Autodesk Fusion 360 part; units mm, degrees
(part 22 of 25)
sketch "Through Holes" plane through (0, 0, 0) normal (0, 0, 1) x (1, 0, 0)
  line L0 (72.5558, 49.13) -> (72.2242, 49.13)
  line L1 (72.2242, 49.13) -> (71.99, 49.3642)
  line L2 (72.7901, 49.6958) -> (72.7901, 49.3642)
  line L3 (72.2242, 49.9301) -> (72.5558, 49.9301)
  line L4 (74.53, 49.6958) -> (74.7642, 49.9301)
  line L5 (71.99, 49.3642) -> (71.99, 49.6958)
  arc A0 (68.1101, 6.35) -> (69.0499, 6.35) centre (68.58, 6.35) ccw
  line L6 (74.7642, 49.13) -> (74.53, 49.3642)
  line L7 (75.0958, 49.13) -> (74.7642, 49.13)
  line L8 (71.99, 49.6958) -> (72.2242, 49.9301)
  line L9 (74.7642, 49.9301) -> (75.0958, 49.9301)
  line L10 (72.2242, 49.9301) -> (72.5558, 49.9301)
  line L11 (74.53, 49.3642) -> (74.53, 49.6958)
  line L12 (75.0958, 49.13) -> (74.7642, 49.13)
  line L13 (75.3301, 49.3642) -> (75.0958, 49.13)
  line L14 (72.5558, 49.9301) -> (72.7901, 49.6958)
  arc A1 (66.5099, 6.35) -> (65.5701, 6.35) centre (66.04, 6.35) ccw
  line L15 (72.7901, 49.3642) -> (72.5558, 49.13)
  line L16 (74.7642, 49.9301) -> (75.0958, 49.9301)
  line L17 (74.7642, 49.13) -> (74.53, 49.3642)
  line L18 (72.7901, 49.3642) -> (72.5558, 49.13)
  line L19 (72.2242, 49.13) -> (71.99, 49.3642)
  line L20 (71.99, 49.3642) -> (71.99, 49.6958)
  line L21 (74.53, 49.6958) -> (74.7642, 49.9301)
  line L22 (71.99, 49.3642) -> (71.99, 49.6958)
  line L23 (75.3301, 49.3642) -> (75.0958, 49.13)
  line L24 (53.1558, 17.3355) -> (52.8955, 17.5958)
  line L25 (53.7845, 17.5958) -> (53.5242, 17.3355)
  arc A2 (50.8, 18.2245) -> (50.8, 17.3355) centre (50.8, 17.78) ccw
  line L26 (53.5242, 17.3355) -> (53.1558, 17.3355)
  line L27 (74.53, 49.3642) -> (74.53, 49.6958)
  arc A3 (50.8, 17.3355) -> (50.8, 18.2245) centre (50.8, 17.78) ccw
  line L28 (53.1558, 18.2245) -> (53.5242, 18.2245)
  arc A4 (50.8, 18.2245) -> (50.8, 17.3355) centre (50.8, 17.78) ccw
  line L29 (72.7901, 49.6958) -> (72.7901, 49.3642)
  line L30 (75.3301, 49.6958) -> (75.3301, 49.3642)
  line L31 (53.5242, 18.2245) -> (53.7845, 17.9642)
  line L32 (52.8955, 17.5958) -> (52.8955, 17.9642)
  line L33 (52.8955, 17.9642) -> (53.1558, 18.2245)
  arc A5 (65.5701, 6.35) -> (66.5099, 6.35) centre (66.04, 6.35) ccw
  line L34 (74.53, 49.3642) -> (74.53, 49.6958)
  arc A6 (69.0499, 6.35) -> (68.1101, 6.35) centre (68.58, 6.35) ccw
  line L35 (74.53, 49.3642) -> (74.53, 49.6958)
  line L36 (72.5558, 49.13) -> (72.2242, 49.13)
  line L37 (75.3301, 49.6958) -> (75.3301, 49.3642)
  line L38 (71.99, 49.6958) -> (72.2242, 49.9301)
  line L39 (72.5558, 49.9301) -> (72.7901, 49.6958)
  line L40 (52.8955, 17.5958) -> (52.8955, 17.9642)
  line L41 (75.0958, 49.9301) -> (75.3301, 49.6958)
  line L42 (75.0958, 49.9301) -> (75.3301, 49.6958)
  line L43 (71.99, 49.3642) -> (71.99, 49.6958)
  arc A7 (61.4299, 6.35) -> (60.4901, 6.35) centre (60.96, 6.35) ccw
  arc A8 (40.1701, 6.35) -> (41.1099, 6.35) centre (40.64, 6.35) ccw
  arc A9 (57.9501, 6.35) -> (58.8899, 6.35) centre (58.42, 6.35) ccw
  arc A10 (14.3891, 33.909) -> (13.5509, 33.909) centre (13.97, 33.909) ccw
  arc A11 (4.318, 50.3555) -> (4.318, 53.5305) centre (4.318, 51.943) ccw
  arc A12 (14.3891, 44.069) -> (13.5509, 44.069) centre (13.97, 44.069) ccw
  arc A13 (50.8, 17.3355) -> (50.8, 18.2245) centre (50.8, 17.78) ccw
  arc A14 (33.4899, 6.35) -> (32.5501, 6.35) centre (33.02, 6.35) ccw
  arc A15 (50.3301, 6.35) -> (51.2699, 6.35) centre (50.8, 6.35) ccw
  arc A16 (41.1099, 6.35) -> (40.1701, 6.35) centre (40.64, 6.35) ccw
  arc A17 (45.2501, 6.35) -> (46.1899, 6.35) centre (45.72, 6.35) ccw
  arc A18 (61.4299, 6.35) -> (60.4901, 6.35) centre (60.96, 6.35) ccw
  arc A19 (4.318, 50.3555) -> (4.318, 53.5305) centre (4.318, 51.943) ccw
  arc A20 (45.2501, 6.35) -> (46.1899, 6.35) centre (45.72, 6.35) ccw
  arc A21 (40.1701, 6.35) -> (41.1099, 6.35) centre (40.64, 6.35) ccw
  arc A22 (63.9699, 6.35) -> (63.0301, 6.35) centre (63.5, 6.35) ccw
  arc A23 (66.5099, 6.35) -> (65.5701, 6.35) centre (66.04, 6.35) ccw
  arc A24 (13.5509, 33.909) -> (14.3891, 33.909) centre (13.97, 33.909) ccw
  arc A25 (14.3891, 44.069) -> (13.5509, 44.069) centre (13.97, 44.069) ccw
  arc A26 (80.645, 50.3555) -> (80.645, 53.5305) centre (80.645, 51.943) ccw
  arc A27 (58.8899, 6.35) -> (57.9501, 6.35) centre (58.42, 6.35) ccw
  arc A28 (68.1101, 6.35) -> (69.0499, 6.35) centre (68.58, 6.35) ccw
  arc A29 (37.6301, 6.35) -> (38.5699, 6.35) centre (38.1, 6.35) ccw
  arc A30 (35.0901, 6.35) -> (36.0299, 6.35) centre (35.56, 6.35) ccw
  line L44 (53.1558, 18.2245) -> (53.5242, 18.2245)
  arc A31 (14.3891, 33.909) -> (13.5509, 33.909) centre (13.97, 33.909) ccw
  arc A32 (13.5509, 44.069) -> (14.3891, 44.069) centre (13.97, 44.069) ccw
  arc A33 (32.5501, 6.35) -> (33.4899, 6.35) centre (33.02, 6.35) ccw
  arc A34 (50.3301, 6.35) -> (51.2699, 6.35) centre (50.8, 6.35) ccw
  line L45 (53.7845, 17.5958) -> (53.5242, 17.3355)
  arc A35 (38.5699, 6.35) -> (37.6301, 6.35) centre (38.1, 6.35) ccw
  arc A36 (4.318, 53.5305) -> (4.318, 50.3555) centre (4.318, 51.943) ccw
  arc A37 (43.6499, 6.35) -> (42.7101, 6.35) centre (43.18, 6.35) ccw
  arc A38 (60.4901, 6.35) -> (61.4299, 6.35) centre (60.96, 6.35) ccw
  arc A39 (56.3499, 6.35) -> (55.4101, 6.35) centre (55.88, 6.35) ccw
  arc A40 (69.0499, 6.35) -> (68.1101, 6.35) centre (68.58, 6.35) ccw
  line L46 (52.8955, 17.5958) -> (52.8955, 17.9642)
  arc A41 (13.5509, 33.909) -> (14.3891, 33.909) centre (13.97, 33.909) ccw
  arc A42 (47.7901, 6.35) -> (48.7299, 6.35) centre (48.26, 6.35) ccw
  line L47 (53.5242, 17.3355) -> (53.1558, 17.3355)
  arc A43 (65.5701, 6.35) -> (66.5099, 6.35) centre (66.04, 6.35) ccw
  arc A44 (42.7101, 6.35) -> (43.6499, 6.35) centre (43.18, 6.35) ccw
  arc A45 (63.0301, 6.35) -> (63.9699, 6.35) centre (63.5, 6.35) ccw
  arc A46 (80.645, 53.5305) -> (80.645, 50.3555) centre (80.645, 51.943) ccw
  line L48 (53.7845, 17.9642) -> (53.7845, 17.5958)
  arc A47 (42.7101, 6.35) -> (43.6499, 6.35) centre (43.18, 6.35) ccw
  arc A48 (38.5699, 6.35) -> (37.6301, 6.35) centre (38.1, 6.35) ccw
  arc A49 (56.3499, 6.35) -> (55.4101, 6.35) centre (55.88, 6.35) ccw
  line L49 (52.8955, 17.5958) -> (52.8955, 17.9642)
  arc A50 (4.318, 53.5305) -> (4.318, 50.3555) centre (4.318, 51.943) ccw
  arc A51 (80.645, 50.3555) -> (80.645, 53.5305) centre (80.645, 51.943) ccw
  arc A52 (48.7299, 6.35) -> (47.7901, 6.35) centre (48.26, 6.35) ccw
  arc A53 (33.4899, 6.35) -> (32.5501, 6.35) centre (33.02, 6.35) ccw
  line L50 (52.8955, 17.9642) -> (53.1558, 18.2245)
  arc A54 (36.0299, 6.35) -> (35.0901, 6.35) centre (35.56, 6.35) ccw
  line L51 (53.1558, 17.3355) -> (52.8955, 17.5958)
  arc A55 (32.5501, 6.35) -> (33.4899, 6.35) centre (33.02, 6.35) ccw
  arc A56 (13.5509, 44.069) -> (14.3891, 44.069) centre (13.97, 44.069) ccw
  arc A57 (51.2699, 6.35) -> (50.3301, 6.35) centre (50.8, 6.35) ccw
  arc A58 (43.6499, 6.35) -> (42.7101, 6.35) centre (43.18, 6.35) ccw
  arc A59 (37.6301, 6.35) -> (38.5699, 6.35) centre (38.1, 6.35) ccw
  line L52 (53.5242, 18.2245) -> (53.7845, 17.9642)
  line L53 (53.7845, 17.9642) -> (53.7845, 17.5958)
  arc A60 (80.645, 53.5305) -> (80.645, 50.3555) centre (80.645, 51.943) ccw
  line L54 (40.7768, 32.6898) -> (40.5032, 32.6898)
  line L55 (50.4698, 32.8832) -> (50.4698, 33.1568)
  line L56 (40.3098, 32.8832) -> (40.3098, 33.1568)
  line L57 (40.9702, 32.8832) -> (40.7768, 32.6898)
  line L58 (51.1302, 33.1568) -> (51.1302, 32.8832)
  line L59 (40.9702, 32.8832) -> (40.7768, 32.6898)
  arc A61 (57.9501, 6.35) -> (58.8899, 6.35) centre (58.42, 6.35) ccw
  arc A62 (60.4901, 6.35) -> (61.4299, 6.35) centre (60.96, 6.35) ccw
  line L60 (51.1302, 32.8832) -> (50.9368, 32.6898)
  line L61 (50.6632, 32.6898) -> (50.4698, 32.8832)
  line L62 (40.5032, 32.6898) -> (40.3098, 32.8832)
  line L63 (50.4698, 33.1568) -> (50.6632, 33.3502)
  line L64 (50.6632, 33.3502) -> (50.9368, 33.3502)
  line L65 (50.9368, 33.3502) -> (51.1302, 33.1568)
  line L66 (51.1302, 33.1568) -> (51.1302, 32.8832)
  line L67 (40.3098, 33.1568) -> (40.5032, 33.3502)
  arc A63 (56.3499, 49.53) -> (55.4101, 49.53) centre (55.88, 49.53) ccw
  arc A64 (47.7901, 6.35) -> (48.7299, 6.35) centre (48.26, 6.35) ccw
  arc A65 (63.9699, 6.35) -> (63.0301, 6.35) centre (63.5, 6.35) ccw
  arc A66 (61.4299, 49.53) -> (60.4901, 49.53) centre (60.96, 49.53) ccw
  arc A67 (57.9501, 49.53) -> (58.8899, 49.53) centre (58.42, 49.53) ccw
  arc A68 (55.4101, 49.53) -> (56.3499, 49.53) centre (55.88, 49.53) ccw
  line L68 (40.9702, 33.1568) -> (40.9702, 32.8832)
  arc A69 (53.8099, 6.35) -> (52.8701, 6.35) centre (53.34, 6.35) ccw
  line L69 (40.5032, 32.6898) -> (40.3098, 32.8832)
  arc A70 (55.4101, 6.35) -> (56.3499, 6.35) centre (55.88, 6.35) ccw
  arc A71 (60.4901, 49.53) -> (61.4299, 49.53) centre (60.96, 49.53) ccw
  arc A72 (46.1899, 6.35) -> (45.2501, 6.35) centre (45.72, 6.35) ccw
  arc A73 (58.8899, 49.53) -> (57.9501, 49.53) centre (58.42, 49.53) ccw
  line L70 (50.9368, 32.6898) -> (50.6632, 32.6898)
  line L71 (40.9702, 33.1568) -> (40.9702, 32.8832)
  arc A74 (36.0299, 6.35) -> (35.0901, 6.35) centre (35.56, 6.35) ccw
  arc A75 (55.4101, 49.53) -> (56.3499, 49.53) centre (55.88, 49.53) ccw
  arc A76 (53.8099, 49.53) -> (52.8701, 49.53) centre (53.34, 49.53) ccw
  arc A77 (35.0901, 6.35) -> (36.0299, 6.35) centre (35.56, 6.35) ccw
  line L72 (40.5032, 33.3502) -> (40.7768, 33.3502)
  arc A78 (48.7299, 6.35) -> (47.7901, 6.35) centre (48.26, 6.35) ccw
  line L73 (50.6632, 32.6898) -> (50.4698, 32.8832)
  line L74 (40.3098, 32.8832) -> (40.3098, 33.1568)
  arc A79 (52.8701, 6.35) -> (53.8099, 6.35) centre (53.34, 6.35) ccw
  line L75 (50.4698, 33.1568) -> (50.6632, 33.3502)
  arc A80 (58.8899, 6.35) -> (57.9501, 6.35) centre (58.42, 6.35) ccw
  line L76 (40.5032, 33.3502) -> (40.7768, 33.3502)
  line L77 (40.3098, 33.1568) -> (40.5032, 33.3502)
  line L78 (40.9702, 33.1568) -> (40.9702, 32.8832)
  line L79 (40.7768, 33.3502) -> (40.9702, 33.1568)
  line L80 (40.7768, 33.3502) -> (40.9702, 33.1568)
  line L81 (40.7768, 32.6898) -> (40.5032, 32.6898)
  arc A81 (46.1899, 6.35) -> (45.2501, 6.35) centre (45.72, 6.35) ccw
  line L82 (50.6632, 33.3502) -> (50.9368, 33.3502)
  arc A82 (55.4101, 6.35) -> (56.3499, 6.35) centre (55.88, 6.35) ccw
  arc A83 (41.1099, 6.35) -> (40.1701, 6.35) centre (40.64, 6.35) ccw
  arc A84 (52.8701, 6.35) -> (53.8099, 6.35) centre (53.34, 6.35) ccw
  line L83 (50.9368, 33.3502) -> (51.1302, 33.1568)
  line L84 (51.1302, 32.8832) -> (50.9368, 32.6898)
  arc A85 (53.8099, 6.35) -> (52.8701, 6.35) centre (53.34, 6.35) ccw
  line L85 (51.1302, 33.1568) -> (51.1302, 32.8832)
  line L86 (51.1302, 33.1568) -> (51.1302, 32.8832)
  line L87 (40.9702, 33.1568) -> (40.9702, 32.8832)
  arc A86 (51.2699, 6.35) -> (50.3301, 6.35) centre (50.8, 6.35) ccw
  arc A87 (63.0301, 6.35) -> (63.9699, 6.35) centre (63.5, 6.35) ccw
  line L88 (50.9368, 32.6898) -> (50.6632, 32.6898)
  line L89 (50.4698, 32.8832) -> (50.4698, 33.1568)
  arc A88 (42.7101, 49.53) -> (43.6499, 49.53) centre (43.18, 49.53) ccw
  arc A89 (24.9301, 49.53) -> (25.8699, 49.53) centre (25.4, 49.53) ccw
  arc A90 (28.7401, 24.4602) -> (29.6799, 24.4602) centre (29.21, 24.4602) ccw
  arc A91 (51.2699, 49.53) -> (50.3301, 49.53) centre (50.8, 49.53) ccw
  arc A92 (33.8201, 24.4602) -> (34.7599, 24.4602) centre (34.29, 24.4602) ccw
  line L90 (29.21, 24.4602) -> (29.21, 26.3398)
  line L91 (36.83, 24.4602) -> (36.83, 26.3398)
  arc A93 (28.4099, 49.53) -> (27.4701, 49.53) centre (27.94, 49.53) ccw
  arc A94 (46.1899, 49.53) -> (45.2501, 49.53) centre (45.72, 49.53) ccw
  arc A95 (52.8701, 49.53) -> (53.8099, 49.53) centre (53.34, 49.53) ccw
  line L92 (34.29, 24.4602) -> (34.29, 26.3398)
  line L93 (31.75, 24.4602) -> (31.75, 26.3398)
  arc A96 (60.4901, 49.53) -> (61.4299, 49.53) centre (60.96, 49.53) ccw
  arc A97 (51.2699, 49.53) -> (50.3301, 49.53) centre (50.8, 49.53) ccw
  arc A98 (37.6301, 49.53) -> (38.5699, 49.53) centre (38.1, 49.53) ccw
  arc A99 (38.5699, 49.53) -> (37.6301, 49.53) centre (38.1, 49.53) ccw
  arc A100 (26.2001, 24.4602) -> (27.1399, 24.4602) centre (26.67, 24.4602) ccw
  arc A101 (30.9499, 49.53) -> (30.0101, 49.53) centre (30.48, 49.53) ccw
  arc A102 (24.9301, 49.53) -> (25.8699, 49.53) centre (25.4, 49.53) ccw
  arc A103 (48.7299, 49.53) -> (47.7901, 49.53) centre (48.26, 49.53) ccw
  arc A104 (32.5501, 49.53) -> (33.4899, 49.53) centre (33.02, 49.53) ccw
  arc A105 (25.8699, 49.53) -> (24.9301, 49.53) centre (25.4, 49.53) ccw
  arc A106 (37.6301, 49.53) -> (38.5699, 49.53) centre (38.1, 49.53) ccw
  arc A107 (30.0101, 49.53) -> (30.9499, 49.53) centre (30.48, 49.53) ccw
  arc A108 (45.2501, 49.53) -> (46.1899, 49.53) centre (45.72, 49.53) ccw
  arc A109 (43.6499, 49.53) -> (42.7101, 49.53) centre (43.18, 49.53) ccw
  arc A110 (41.1099, 49.53) -> (40.1701, 49.53) centre (40.64, 49.53) ccw
  arc A111 (50.3301, 49.53) -> (51.2699, 49.53) centre (50.8, 49.53) ccw
  arc A112 (48.7299, 49.53) -> (47.7901, 49.53) centre (48.26, 49.53) ccw
  arc A113 (57.9501, 49.53) -> (58.8899, 49.53) centre (58.42, 49.53) ccw
  arc A114 (25.8699, 49.53) -> (24.9301, 49.53) centre (25.4, 49.53) ccw
  arc A115 (43.6499, 49.53) -> (42.7101, 49.53) centre (43.18, 49.53) ccw
  arc A116 (47.7901, 49.53) -> (48.7299, 49.53) centre (48.26, 49.53) ccw
  arc A117 (56.3499, 49.53) -> (55.4101, 49.53) centre (55.88, 49.53) ccw
  arc A118 (28.4099, 49.53) -> (27.4701, 49.53) centre (27.94, 49.53) ccw
  arc A119 (27.4701, 49.53) -> (28.4099, 49.53) centre (27.94, 49.53) ccw
  arc A120 (46.1899, 49.53) -> (45.2501, 49.53) centre (45.72, 49.53) ccw
  arc A121 (32.5501, 49.53) -> (33.4899, 49.53) centre (33.02, 49.53) ccw
  arc A122 (45.2501, 49.53) -> (46.1899, 49.53) centre (45.72, 49.53) ccw
  arc A123 (33.4899, 49.53) -> (32.5501, 49.53) centre (33.02, 49.53) ccw
  arc A124 (61.4299, 49.53) -> (60.4901, 49.53) centre (60.96, 49.53) ccw
  arc A125 (30.9499, 49.53) -> (30.0101, 49.53) centre (30.48, 49.53) ccw
  arc A126 (42.7101, 49.53) -> (43.6499, 49.53) centre (43.18, 49.53) ccw
  arc A127 (40.1701, 49.53) -> (41.1099, 49.53) centre (40.64, 49.53) ccw
  arc A128 (30.0101, 49.53) -> (30.9499, 49.53) centre (30.48, 49.53) ccw
  arc A129 (38.5699, 49.53) -> (37.6301, 49.53) centre (38.1, 49.53) ccw
  arc A130 (35.0901, 49.53) -> (36.0299, 49.53) centre (35.56, 49.53) ccw
  arc A131 (41.1099, 49.53) -> (40.1701, 49.53) centre (40.64, 49.53) ccw
  line L94 (26.67, 24.4602) -> (26.67, 26.3398)
  arc A132 (58.8899, 49.53) -> (57.9501, 49.53) centre (58.42, 49.53) ccw
  arc A133 (33.4899, 49.53) -> (32.5501, 49.53) centre (33.02, 49.53) ccw
  arc A134 (53.8099, 49.53) -> (52.8701, 49.53) centre (53.34, 49.53) ccw
  arc A135 (36.0299, 49.53) -> (35.0901, 49.53) centre (35.56, 49.53) ccw
  arc A136 (28.7401, 24.4602) -> (29.6799, 24.4602) centre (29.21, 24.4602) ccw
  line L95 (29.21, 24.4602) -> (29.21, 26.3398)
  arc A137 (47.7901, 49.53) -> (48.7299, 49.53) centre (48.26, 49.53) ccw
  arc A138 (27.4701, 49.53) -> (28.4099, 49.53) centre (27.94, 49.53) ccw
  arc A139 (35.0901, 49.53) -> (36.0299, 49.53) centre (35.56, 49.53) ccw
  arc A140 (36.0299, 49.53) -> (35.0901, 49.53) centre (35.56, 49.53) ccw
  arc A141 (50.3301, 49.53) -> (51.2699, 49.53) centre (50.8, 49.53) ccw
  arc A142 (40.1701, 49.53) -> (41.1099, 49.53) centre (40.64, 49.53) ccw
  arc A143 (34.7599, 26.3398) -> (33.8201, 26.3398) centre (34.29, 26.3398) ccw
  arc A144 (52.8701, 49.53) -> (53.8099, 49.53) centre (53.34, 49.53) ccw
  arc A145 (27.1399, 26.3398) -> (26.2001, 26.3398) centre (26.67, 26.3398) ccw
  arc A146 (27.1399, 26.3398) -> (26.2001, 26.3398) centre (26.67, 26.3398) ccw
  arc A147 (36.3601, 24.4602) -> (37.2999, 24.4602) centre (36.83, 24.4602) ccw
  arc A148 (29.6799, 26.3398) -> (28.7401, 26.3398) centre (29.21, 26.3398) ccw
  line L96 (31.75, 24.4602) -> (31.75, 26.3398)
  arc A149 (37.2999, 26.3398) -> (36.3601, 26.3398) centre (36.83, 26.3398) ccw
  arc A150 (29.6799, 26.3398) -> (28.7401, 26.3398) centre (29.21, 26.3398) ccw
  arc A151 (31.2801, 24.4602) -> (32.2199, 24.4602) centre (31.75, 24.4602) ccw
  line L97 (34.29, 24.4602) -> (34.29, 26.3398)
  arc A152 (34.7599, 26.3398) -> (33.8201, 26.3398) centre (34.29, 26.3398) ccw
  arc A153 (26.2001, 24.4602) -> (27.1399, 24.4602) centre (26.67, 24.4602) ccw
  arc A154 (31.2801, 24.4602) -> (32.2199, 24.4602) centre (31.75, 24.4602) ccw
  line L98 (26.67, 24.4602) -> (26.67, 26.3398)
  arc A155 (32.2199, 26.3398) -> (31.2801, 26.3398) centre (31.75, 26.3398) ccw
  arc A156 (37.2999, 26.3398) -> (36.3601, 26.3398) centre (36.83, 26.3398) ccw
  arc A157 (74.1299, 32.6898) -> (73.1901, 32.6898) centre (73.66, 32.6898) ccw
  line L99 (78.74, 43.5102) -> (78.74, 45.3898)
  line L100 (76.2, 30.8102) -> (76.2, 32.6898)
  arc A158 (81.7499, 45.3898) -> (80.8101, 45.3898) centre (81.28, 45.3898) ccw
  arc A159 (79.2099, 45.3898) -> (78.2701, 45.3898) centre (78.74, 45.3898) ccw
  arc A160 (73.1901, 43.5102) -> (74.1299, 43.5102) centre (73.66, 43.5102) ccw
  line L101 (73.66, 43.5102) -> (73.66, 45.3898)
  line L102 (36.83, 24.4602) -> (36.83, 26.3398)
  line L103 (76.2, 43.5102) -> (76.2, 45.3898)
  arc A161 (81.7499, 45.3898) -> (80.8101, 45.3898) centre (81.28, 45.3898) ccw
  line L104 (78.74, 30.8102) -> (78.74, 32.6898)
  arc A162 (80.8101, 43.5102) -> (81.7499, 43.5102) centre (81.28, 43.5102) ccw
  arc A163 (73.1901, 30.8102) -> (74.1299, 30.8102) centre (73.66, 30.8102) ccw
  arc A164 (33.8201, 24.4602) -> (34.7599, 24.4602) centre (34.29, 24.4602) ccw
  arc A165 (79.2099, 45.3898) -> (78.2701, 45.3898) centre (78.74, 45.3898) ccw
  arc A166 (76.6699, 45.3898) -> (75.7301, 45.3898) centre (76.2, 45.3898) ccw
  arc A167 (76.6699, 45.3898) -> (75.7301, 45.3898) centre (76.2, 45.3898) ccw
  line L105 (73.66, 30.8102) -> (73.66, 32.6898)
  arc A168 (75.7301, 30.8102) -> (76.6699, 30.8102) centre (76.2, 30.8102) ccw
  line L106 (81.28, 43.5102) -> (81.28, 45.3898)
  line L107 (73.66, 30.8102) -> (73.66, 32.6898)
  arc A169 (74.1299, 45.3898) -> (73.1901, 45.3898) centre (73.66, 45.3898) ccw
  line L108 (73.66, 43.5102) -> (73.66, 45.3898)
  arc A170 (76.6699, 32.6898) -> (75.7301, 32.6898) centre (76.2, 32.6898) ccw
  arc A171 (75.7301, 30.8102) -> (76.6699, 30.8102) centre (76.2, 30.8102) ccw
  arc A172 (73.1901, 30.8102) -> (74.1299, 30.8102) centre (73.66, 30.8102) ccw
  arc A173 (78.2701, 43.5102) -> (79.2099, 43.5102) centre (78.74, 43.5102) ccw
  arc A174 (76.6699, 32.6898) -> (75.7301, 32.6898) centre (76.2, 32.6898) ccw
  arc A175 (74.1299, 45.3898) -> (73.1901, 45.3898) centre (73.66, 45.3898) ccw
  arc A176 (75.7301, 43.5102) -> (76.6699, 43.5102) centre (76.2, 43.5102) ccw
  arc A177 (75.7301, 43.5102) -> (76.6699, 43.5102) centre (76.2, 43.5102) ccw
  line L109 (76.2, 30.8102) -> (76.2, 32.6898)
  arc A178 (80.8101, 43.5102) -> (81.7499, 43.5102) centre (81.28, 43.5102) ccw
  arc A179 (36.3601, 24.4602) -> (37.2999, 24.4602) centre (36.83, 24.4602) ccw
  line L110 (81.28, 43.5102) -> (81.28, 45.3898)
  arc A180 (74.1299, 32.6898) -> (73.1901, 32.6898) centre (73.66, 32.6898) ccw
  arc A181 (78.2701, 43.5102) -> (79.2099, 43.5102) centre (78.74, 43.5102) ccw
  arc A182 (73.1901, 43.5102) -> (74.1299, 43.5102) centre (73.66, 43.5102) ccw
  arc A183 (32.2199, 26.3398) -> (31.2801, 26.3398) centre (31.75, 26.3398) ccw
  line L111 (78.74, 43.5102) -> (78.74, 45.3898)
  line L112 (76.2, 43.5102) -> (76.2, 45.3898)
  line L113 (63.5, 42.2402) -> (63.5, 44.1198)
  arc A184 (58.8899, 44.1198) -> (57.9501, 44.1198) centre (58.42, 44.1198) ccw
  line L114 (27.0701, 37.9342) -> (26.8358, 37.7)
  arc A185 (65.5701, 42.2402) -> (66.5099, 42.2402) centre (66.04, 42.2402) ccw
  line L115 (34.4558, 37.7) -> (34.1242, 37.7)
  line L116 (26.5042, 37.7) -> (26.27, 37.9342)
  arc A186 (81.7499, 32.6898) -> (80.8101, 32.6898) centre (81.28, 32.6898) ccw
  line L117 (66.04, 42.2402) -> (66.04, 44.1198)
  line L118 (63.5, 42.2402) -> (63.5, 44.1198)
  arc A187 (60.4901, 42.2402) -> (61.4299, 42.2402) centre (60.96, 42.2402) ccw
  arc A188 (66.5099, 44.1198) -> (65.5701, 44.1198) centre (66.04, 44.1198) ccw
  line L119 (33.89, 37.9342) -> (33.89, 38.2658)
  line L120 (34.1242, 37.7) -> (33.89, 37.9342)
  line L121 (34.69, 38.2658) -> (34.69, 37.9342)
  line L122 (34.69, 37.9342) -> (34.4558, 37.7)
  line L123 (34.4558, 37.7) -> (34.1242, 37.7)
  line L124 (34.69, 38.2658) -> (34.69, 37.9342)
  line L125 (34.1242, 38.5001) -> (34.4558, 38.5001)
  arc A189 (63.9699, 44.1198) -> (63.0301, 44.1198) centre (63.5, 44.1198) ccw
  line L126 (81.28, 30.8102) -> (81.28, 32.6898)
  arc A190 (80.8101, 30.8102) -> (81.7499, 30.8102) centre (81.28, 30.8102) ccw
  arc A191 (65.5701, 42.2402) -> (66.5099, 42.2402) centre (66.04, 42.2402) ccw
  arc A192 (65.5701, 30.8102) -> (66.5099, 30.8102) centre (66.04, 30.8102) ccw
  arc A193 (61.4299, 32.6898) -> (60.4901, 32.6898) centre (60.96, 32.6898) ccw
  line L127 (66.04, 42.2402) -> (66.04, 44.1198)
  arc A194 (63.9699, 44.1198) -> (63.0301, 44.1198) centre (63.5, 44.1198) ccw
  arc A195 (63.0301, 42.2402) -> (63.9699, 42.2402) centre (63.5, 42.2402) ccw
  arc A196 (79.2099, 32.6898) -> (78.2701, 32.6898) centre (78.74, 32.6898) ccw
  line L128 (26.8358, 37.7) -> (26.5042, 37.7)
  arc A197 (81.7499, 32.6898) -> (80.8101, 32.6898) centre (81.28, 32.6898) ccw
  arc A198 (63.0301, 30.8102) -> (63.9699, 30.8102) centre (63.5, 30.8102) ccw
  line L129 (34.69, 38.2658) -> (34.69, 37.9342)
  line L130 (34.4558, 38.5001) -> (34.69, 38.2658)
  arc A199 (60.4901, 42.2402) -> (61.4299, 42.2402) centre (60.96, 42.2402) ccw
  arc A200 (63.0301, 30.8102) -> (63.9699, 30.8102) centre (63.5, 30.8102) ccw
  arc A201 (61.4299, 44.1198) -> (60.4901, 44.1198) centre (60.96, 44.1198) ccw
  arc A202 (79.2099, 32.6898) -> (78.2701, 32.6898) centre (78.74, 32.6898) ccw
  line L131 (26.5042, 38.5001) -> (26.8358, 38.5001)
  line L132 (60.96, 42.2402) -> (60.96, 44.1198)
  arc A203 (57.9501, 42.2402) -> (58.8899, 42.2402) centre (58.42, 42.2402) ccw
  arc A204 (61.4299, 44.1198) -> (60.4901, 44.1198) centre (60.96, 44.1198) ccw
  line L133 (33.89, 38.2658) -> (34.1242, 38.5001)
  arc A205 (58.8899, 44.1198) -> (57.9501, 44.1198) centre (58.42, 44.1198) ccw
  line L134 (58.42, 42.2402) -> (58.42, 44.1198)
  line L135 (26.27, 37.9342) -> (26.27, 38.2658)
  line L136 (33.89, 38.2658) -> (34.1242, 38.5001)
  line L137 (34.69, 37.9342) -> (34.4558, 37.7)
  line L138 (33.89, 37.9342) -> (33.89, 38.2658)
  line L139 (81.28, 30.8102) -> (81.28, 32.6898)
  line L140 (58.42, 42.2402) -> (58.42, 44.1198)
  line L141 (27.0701, 38.2658) -> (27.0701, 37.9342)
  line L142 (60.96, 42.2402) -> (60.96, 44.1198)
  arc A206 (80.8101, 30.8102) -> (81.7499, 30.8102) centre (81.28, 30.8102) ccw
  line L143 (26.8358, 37.7) -> (26.5042, 37.7)
  arc A207 (63.0301, 42.2402) -> (63.9699, 42.2402) centre (63.5, 42.2402) ccw
  line L144 (34.4558, 38.5001) -> (34.69, 38.2658)
  line L145 (34.1242, 38.5001) -> (34.4558, 38.5001)
  arc A208 (78.2701, 30.8102) -> (79.2099, 30.8102) centre (78.74, 30.8102) ccw
  line L146 (26.27, 38.2658) -> (26.5042, 38.5001)
  arc A209 (57.9501, 42.2402) -> (58.8899, 42.2402) centre (58.42, 42.2402) ccw
  line L147 (34.1242, 37.7) -> (33.89, 37.9342)
  arc A210 (78.2701, 30.8102) -> (79.2099, 30.8102) centre (78.74, 30.8102) ccw
  line L148 (78.74, 30.8102) -> (78.74, 32.6898)
  arc A211 (66.5099, 44.1198) -> (65.5701, 44.1198) centre (66.04, 44.1198) ccw
  line L149 (34.69, 38.2658) -> (34.69, 37.9342)
  arc A212 (16.9799, 50.4698) -> (16.0401, 50.4698) centre (16.51, 50.4698) ccw
  line L150 (26.5042, 38.5001) -> (26.8358, 38.5001)
  arc A213 (61.4299, 32.6898) -> (60.4901, 32.6898) centre (60.96, 32.6898) ccw
  arc A214 (11.8999, 50.4698) -> (10.9601, 50.4698) centre (11.43, 50.4698) ccw
  line L151 (26.27, 37.9342) -> (26.27, 38.2658)
  line L152 (26.8358, 38.5001) -> (27.0701, 38.2658)
  arc A215 (65.5701, 30.8102) -> (66.5099, 30.8102) centre (66.04, 30.8102) ccw
  line L153 (27.0701, 38.2658) -> (27.0701, 37.9342)
  line L154 (60.96, 32.6898) -> (60.96, 30.8102)
  arc A216 (66.5099, 32.6898) -> (65.5701, 32.6898) centre (66.04, 32.6898) ccw
  line L155 (63.5, 32.6898) -> (63.5, 30.8102)
  arc A217 (19.5199, 50.4698) -> (18.5801, 50.4698) centre (19.05, 50.4698) ccw
  arc A218 (66.5099, 32.6898) -> (65.5701, 32.6898) centre (66.04, 32.6898) ccw
  line L156 (16.51, 50.4698) -> (16.51, 48.5902)
  line L157 (21.59, 50.4698) -> (21.59, 48.5902)
  arc A219 (13.5001, 48.5902) -> (14.4399, 48.5902) centre (13.97, 48.5902) ccw
  arc A220 (60.4901, 30.8102) -> (61.4299, 30.8102) centre (60.96, 30.8102) ccw
  line L158 (11.43, 50.4698) -> (11.43, 48.5902)
  line L159 (19.05, 50.4698) -> (19.05, 48.5902)
  arc A221 (14.4399, 50.4698) -> (13.5001, 50.4698) centre (13.97, 50.4698) ccw
  arc A222 (11.8999, 50.4698) -> (10.9601, 50.4698) centre (11.43, 50.4698) ccw
  line L160 (27.0701, 37.9342) -> (26.8358, 37.7)
  line L161 (66.04, 32.6898) -> (66.04, 30.8102)
  line L162 (26.8358, 38.5001) -> (27.0701, 38.2658)
  line L163 (13.97, 50.4698) -> (13.97, 48.5902)
  arc A223 (60.4901, 30.8102) -> (61.4299, 30.8102) centre (60.96, 30.8102) ccw
  arc A224 (22.0599, 50.4698) -> (21.1201, 50.4698) centre (21.59, 50.4698) ccw
  arc A225 (18.5801, 48.5902) -> (19.5199, 48.5902) centre (19.05, 48.5902) ccw
  arc A226 (13.5001, 48.5902) -> (14.4399, 48.5902) centre (13.97, 48.5902) ccw
  line L164 (11.43, 50.4698) -> (11.43, 48.5902)
  line L165 (26.5042, 34.69) -> (26.8358, 34.69)
  line L166 (34.69, 34.4558) -> (34.69, 34.1242)
  line L167 (26.8358, 34.69) -> (27.0701, 34.4558)
  arc A227 (21.1201, 48.5902) -> (22.0599, 48.5902) centre (21.59, 48.5902) ccw
  line L168 (26.27, 38.2658) -> (26.5042, 38.5001)
  arc A228 (21.1201, 48.5902) -> (22.0599, 48.5902) centre (21.59, 48.5902) ccw
  line L169 (13.97, 50.4698) -> (13.97, 48.5902)
  line L170 (19.05, 50.4698) -> (19.05, 48.5902)
  line L171 (27.0701, 34.4558) -> (27.0701, 34.1242)
  line L172 (26.27, 34.1242) -> (26.27, 34.4558)
  arc A229 (63.9699, 32.6898) -> (63.0301, 32.6898) centre (63.5, 32.6898) ccw
  arc A230 (16.9799, 50.4698) -> (16.0401, 50.4698) centre (16.51, 50.4698) ccw
  line L173 (26.5042, 33.89) -> (26.27, 34.1242)
  line L174 (27.0701, 34.4558) -> (27.0701, 34.1242)
  line L175 (27.0701, 38.2658) -> (27.0701, 37.9342)
  arc A231 (16.0401, 48.5902) -> (16.9799, 48.5902) centre (16.51, 48.5902) ccw
  arc A232 (10.9601, 48.5902) -> (11.8999, 48.5902) centre (11.43, 48.5902) ccw
  arc A233 (14.4399, 50.4698) -> (13.5001, 50.4698) centre (13.97, 50.4698) ccw
  line L176 (34.4558, 33.89) -> (34.1242, 33.89)
  line L177 (21.59, 50.4698) -> (21.59, 48.5902)
  line L178 (27.0701, 38.2658) -> (27.0701, 37.9342)
  arc A234 (19.5199, 50.4698) -> (18.5801, 50.4698) centre (19.05, 50.4698) ccw
  line L179 (60.96, 32.6898) -> (60.96, 30.8102)
  arc A235 (63.9699, 32.6898) -> (63.0301, 32.6898) centre (63.5, 32.6898) ccw
  arc A236 (16.0401, 48.5902) -> (16.9799, 48.5902) centre (16.51, 48.5902) ccw
  line L180 (63.5, 32.6898) -> (63.5, 30.8102)
  line L181 (34.4558, 33.89) -> (34.1242, 33.89)
  line L182 (34.69, 34.1242) -> (34.4558, 33.89)
  line L183 (26.5042, 37.7) -> (26.27, 37.9342)
  arc A237 (22.0599, 50.4698) -> (21.1201, 50.4698) centre (21.59, 50.4698) ccw
  arc A238 (10.9601, 48.5902) -> (11.8999, 48.5902) centre (11.43, 48.5902) ccw
  line L184 (66.04, 32.6898) -> (66.04, 30.8102)
  line L185 (16.51, 50.4698) -> (16.51, 48.5902)
  arc A239 (18.5801, 48.5902) -> (19.5199, 48.5902) centre (19.05, 48.5902) ccw
  line L186 (26.5042, 33.89) -> (26.27, 34.1242)
  arc A240 (50.3301, 24.4602) -> (51.2699, 24.4602) centre (50.8, 24.4602) ccw
  line L187 (48.26, 24.4602) -> (48.26, 26.3398)
  arc A241 (25.8699, 16.51) -> (24.9301, 16.51) centre (25.4, 16.51) ccw
  line L188 (34.69, 34.4558) -> (34.69, 34.1242)
  arc A242 (30.9499, 16.51) -> (30.0101, 16.51) centre (30.48, 16.51) ccw
  line L189 (26.8358, 33.89) -> (26.5042, 33.89)
  line L190 (53.34, 24.4602) -> (53.34, 26.3398)
  line L191 (34.1242, 34.69) -> (34.4558, 34.69)
  line L192 (33.89, 34.1242) -> (33.89, 34.4558)
  arc A243 (36.0299, 16.51) -> (35.0901, 16.51) centre (35.56, 16.51) ccw
  arc A244 (27.4701, 16.51) -> (28.4099, 16.51) centre (27.94, 16.51) ccw
  arc A245 (23.3299, 16.51) -> (22.3901, 16.51) centre (22.86, 16.51) ccw
  arc A246 (30.0101, 16.51) -> (30.9499, 16.51) centre (30.48, 16.51) ccw
  line L193 (27.0701, 34.1242) -> (26.8358, 33.89)
  arc A247 (27.4701, 16.51) -> (28.4099, 16.51) centre (27.94, 16.51) ccw
  arc A248 (33.4899, 16.51) -> (32.5501, 16.51) centre (33.02, 16.51) ccw
  arc A249 (51.2699, 26.3398) -> (50.3301, 26.3398) centre (50.8, 26.3398) ccw
  arc A250 (22.3901, 16.51) -> (23.3299, 16.51) centre (22.86, 16.51) ccw
  arc A251 (51.2699, 26.3398) -> (50.3301, 26.3398) centre (50.8, 26.3398) ccw
  line L194 (48.26, 24.4602) -> (48.26, 26.3398)
  arc A252 (47.7901, 24.4602) -> (48.7299, 24.4602) centre (48.26, 24.4602) ccw
  arc A253 (47.7901, 24.4602) -> (48.7299, 24.4602) centre (48.26, 24.4602) ccw
  line L195 (34.69, 34.4558) -> (34.69, 34.1242)
  arc A254 (22.3901, 16.51) -> (23.3299, 16.51) centre (22.86, 16.51) ccw
  line L196 (26.8358, 34.69) -> (27.0701, 34.4558)
  arc A255 (24.9301, 16.51) -> (25.8699, 16.51) centre (25.4, 16.51) ccw
  line L197 (27.0701, 34.4558) -> (27.0701, 34.1242)
  arc A256 (52.8701, 24.4602) -> (53.8099, 24.4602) centre (53.34, 24.4602) ccw
  line L198 (34.1242, 33.89) -> (33.89, 34.1242)
  line L199 (33.89, 34.4558) -> (34.1242, 34.69)
  arc A257 (50.3301, 24.4602) -> (51.2699, 24.4602) centre (50.8, 24.4602) ccw
  arc A258 (48.7299, 26.3398) -> (47.7901, 26.3398) centre (48.26, 26.3398) ccw
  line L200 (50.8, 24.4602) -> (50.8, 26.3398)
  line L201 (26.27, 34.4558) -> (26.5042, 34.69)
  line L202 (53.34, 24.4602) -> (53.34, 26.3398)
  arc A259 (33.4899, 16.51) -> (32.5501, 16.51) centre (33.02, 16.51) ccw
  line L203 (50.8, 24.4602) -> (50.8, 26.3398)
  line L204 (26.8358, 33.89) -> (26.5042, 33.89)
  arc A260 (28.4099, 16.51) -> (27.4701, 16.51) centre (27.94, 16.51) ccw
  line L205 (34.4558, 34.69) -> (34.69, 34.4558)
  line L206 (34.1242, 34.69) -> (34.4558, 34.69)
  line L207 (34.69, 34.1242) -> (34.4558, 33.89)
  arc A261 (23.3299, 16.51) -> (22.3901, 16.51) centre (22.86, 16.51) ccw
  arc A262 (32.5501, 16.51) -> (33.4899, 16.51) centre (33.02, 16.51) ccw
  arc A263 (53.8099, 26.3398) -> (52.8701, 26.3398) centre (53.34, 26.3398) ccw
  line L208 (33.89, 34.1242) -> (33.89, 34.4558)
  line L209 (26.5042, 34.69) -> (26.8358, 34.69)
  line L210 (26.27, 34.1242) -> (26.27, 34.4558)
  arc A264 (48.7299, 26.3398) -> (47.7901, 26.3398) centre (48.26, 26.3398) ccw
  arc A265 (24.9301, 16.51) -> (25.8699, 16.51) centre (25.4, 16.51) ccw
  line L211 (27.0701, 34.4558) -> (27.0701, 34.1242)
  line L212 (34.1242, 33.89) -> (33.89, 34.1242)
  line L213 (34.4558, 34.69) -> (34.69, 34.4558)
  arc A266 (53.8099, 26.3398) -> (52.8701, 26.3398) centre (53.34, 26.3398) ccw
  arc A267 (28.4099, 16.51) -> (27.4701, 16.51) centre (27.94, 16.51) ccw
  arc A268 (52.8701, 24.4602) -> (53.8099, 24.4602) centre (53.34, 24.4602) ccw
  arc A269 (30.9499, 16.51) -> (30.0101, 16.51) centre (30.48, 16.51) ccw
  line L214 (26.27, 34.4558) -> (26.5042, 34.69)
  line L215 (34.69, 34.4558) -> (34.69, 34.1242)
  line L216 (27.0701, 34.1242) -> (26.8358, 33.89)
  line L217 (33.89, 34.4558) -> (34.1242, 34.69)
  arc A270 (25.8699, 16.51) -> (24.9301, 16.51) centre (25.4, 16.51) ccw
  arc A271 (30.0101, 16.51) -> (30.9499, 16.51) centre (30.48, 16.51) ccw
  arc A272 (7.4676, 34.6202) -> (7.4676, 33.9598) centre (7.4676, 34.29) ccw
  arc A273 (2.3876, 34.6202) -> (2.3876, 33.9598) centre (2.3876, 34.29) ccw
  line L218 (7.4676, 41.91) -> (8.7884, 41.91)
  arc A274 (35.0901, 16.51) -> (36.0299, 16.51) centre (35.56, 16.51) ccw
  line L219 (4.8936, 6.7564) -> (5.241, 6.7564)
  arc A275 (3.7084, 44.1198) -> (3.7084, 44.7802) centre (3.7084, 44.45) ccw
  line L220 (2.3876, 44.45) -> (3.7084, 44.45)
  arc A276 (40.1701, 16.51) -> (41.1099, 16.51) centre (40.64, 16.51) ccw
  arc A277 (35.0901, 16.51) -> (36.0299, 16.51) centre (35.56, 16.51) ccw
  arc A278 (3.7084, 33.9598) -> (3.7084, 34.6202) centre (3.7084, 34.29) ccw
  line L221 (7.4676, 44.45) -> (8.7884, 44.45)
  arc A279 (8.7884, 33.9598) -> (8.7884, 34.6202) centre (8.7884, 34.29) ccw
  arc A280 (2.3876, 44.7802) -> (2.3876, 44.1198) centre (2.3876, 44.45) ccw
  arc A281 (32.5501, 16.51) -> (33.4899, 16.51) centre (33.02, 16.51) ccw
  arc A282 (8.7884, 44.1198) -> (8.7884, 44.7802) centre (8.7884, 44.45) ccw
  arc A283 (3.7084, 44.1198) -> (3.7084, 44.7802) centre (3.7084, 44.45) ccw
  arc A284 (8.7884, 41.5798) -> (8.7884, 42.2402) centre (8.7884, 41.91) ccw
  arc A285 (3.7084, 41.5798) -> (3.7084, 42.2402) centre (3.7084, 41.91) ccw
  arc A286 (8.7884, 33.9598) -> (8.7884, 34.6202) centre (8.7884, 34.29) ccw
  arc A287 (2.3876, 42.2402) -> (2.3876, 41.5798) centre (2.3876, 41.91) ccw
  line L222 (4.6482, 3.971) -> (4.8936, 4.2164)
  arc A288 (3.7084, 41.5798) -> (3.7084, 42.2402) centre (3.7084, 41.91) ccw
  line L223 (4.6482, 6.511) -> (4.8936, 6.7564)
  line L224 (2.3876, 41.91) -> (3.7084, 41.91)
  line L225 (7.4676, 44.45) -> (8.7884, 44.45)
  arc A289 (7.4676, 42.2402) -> (7.4676, 41.5798) centre (7.4676, 41.91) ccw
  arc A290 (38.5699, 16.51) -> (37.6301, 16.51) centre (38.1, 16.51) ccw
  line L226 (4.8936, 5.9182) -> (4.6482, 6.1636)
  arc A291 (7.4676, 44.7802) -> (7.4676, 44.1198) centre (7.4676, 44.45) ccw
  line L227 (5.4864, 3.6236) -> (5.241, 3.3782)
  arc A292 (8.7884, 44.1198) -> (8.7884, 44.7802) centre (8.7884, 44.45) ccw
  arc A293 (7.4676, 34.6202) -> (7.4676, 33.9598) centre (7.4676, 34.29) ccw
  arc A294 (7.4676, 42.2402) -> (7.4676, 41.5798) centre (7.4676, 41.91) ccw
  arc A295 (8.7884, 41.5798) -> (8.7884, 42.2402) centre (8.7884, 41.91) ccw
  arc A296 (2.3876, 42.2402) -> (2.3876, 41.5798) centre (2.3876, 41.91) ccw
  line L228 (4.6482, 3.6236) -> (4.6482, 3.971)
  line L229 (5.4864, 3.6236) -> (5.241, 3.3782)
  line L230 (5.4864, 3.971) -> (5.4864, 3.6236)
  line L231 (5.241, 5.9182) -> (4.8936, 5.9182)
  line L232 (2.3876, 41.91) -> (3.7084, 41.91)
  line L233 (5.241, 5.9182) -> (4.8936, 5.9182)
  arc A297 (7.4676, 44.7802) -> (7.4676, 44.1198) centre (7.4676, 44.45) ccw
  line L234 (7.4676, 34.29) -> (8.7884, 34.29)
  line L235 (5.241, 6.7564) -> (5.4864, 6.511)
  line L236 (4.8936, 4.2164) -> (5.241, 4.2164)
  line L237 (4.6482, 6.1636) -> (4.6482, 6.511)
  line L238 (4.8936, 5.9182) -> (4.6482, 6.1636)
  arc A298 (41.1099, 16.51) -> (40.1701, 16.51) centre (40.64, 16.51) ccw
  arc A299 (41.1099, 16.51) -> (40.1701, 16.51) centre (40.64, 16.51) ccw
  arc A300 (2.3876, 44.7802) -> (2.3876, 44.1198) centre (2.3876, 44.45) ccw
  arc A301 (2.3876, 34.6202) -> (2.3876, 33.9598) centre (2.3876, 34.29) ccw
  line L239 (7.4676, 34.29) -> (8.7884, 34.29)
  arc A302 (40.1701, 16.51) -> (41.1099, 16.51) centre (40.64, 16.51) ccw
  arc A303 (3.7084, 33.9598) -> (3.7084, 34.6202) centre (3.7084, 34.29) ccw
  line L240 (5.241, 4.2164) -> (5.4864, 3.971)
  line L241 (2.3876, 44.45) -> (3.7084, 44.45)
  arc A304 (36.0299, 16.51) -> (35.0901, 16.51) centre (35.56, 16.51) ccw
  arc A305 (37.6301, 16.51) -> (38.5699, 16.51) centre (38.1, 16.51) ccw
  arc A306 (37.6301, 16.51) -> (38.5699, 16.51) centre (38.1, 16.51) ccw
  arc A307 (38.5699, 16.51) -> (37.6301, 16.51) centre (38.1, 16.51) ccw
  line L242 (2.3876, 34.29) -> (3.7084, 34.29)
  line L243 (2.3876, 34.29) -> (3.7084, 34.29)
  line L244 (4.8936, 6.7564) -> (5.241, 6.7564)
  line L245 (7.4676, 41.91) -> (8.7884, 41.91)
  line L246 (13.5509, 3.9837) -> (13.7963, 4.2291)
  line L247 (4.8936, 3.3782) -> (4.6482, 3.6236)
  line L248 (72.1868, 12.3092) -> (72.1868, 12.5828)
  line L249 (14.1437, 4.2291) -> (14.3891, 3.9837)
  line L250 (72.6538, 12.7762) -> (72.8472, 12.5828)
  line L251 (14.1437, 6.7691) -> (14.3891, 6.5237)
  line L252 (4.8936, 4.2164) -> (5.241, 4.2164)
  line L253 (14.1437, 5.9309) -> (13.7963, 5.9309)
  line L254 (5.4864, 6.1636) -> (5.241, 5.9182)
  line L255 (5.4864, 6.511) -> (5.4864, 6.1636)
  line L256 (13.5509, 6.5237) -> (13.7963, 6.7691)
  line L257 (13.5509, 6.1763) -> (13.5509, 6.5237)
  line L258 (14.3891, 3.6363) -> (14.1437, 3.3909)
  line L259 (72.3802, 12.7762) -> (72.6538, 12.7762)
  line L260 (5.241, 4.2164) -> (5.4864, 3.971)
  line L261 (4.6482, 3.971) -> (4.8936, 4.2164)
  line L262 (4.6482, 6.1636) -> (4.6482, 6.511)
  line L263 (13.7963, 4.2291) -> (14.1437, 4.2291)
  line L264 (14.3891, 6.1763) -> (14.1437, 5.9309)
  line L265 (14.1437, 3.3909) -> (13.7963, 3.3909)
  line L266 (72.6538, 12.7762) -> (72.8472, 12.5828)
  line L267 (5.241, 3.3782) -> (4.8936, 3.3782)
  line L268 (72.8472, 12.5828) -> (72.8472, 12.3092)
  line L269 (13.5509, 3.9837) -> (13.7963, 4.2291)
  line L270 (5.4864, 6.511) -> (5.4864, 6.1636)
  line L271 (4.8936, 3.3782) -> (4.6482, 3.6236)
  line L272 (4.6482, 3.6236) -> (4.6482, 3.971)
  line L273 (4.8936, 4.2164) -> (5.241, 4.2164)
  line L274 (13.7963, 6.7691) -> (14.1437, 6.7691)
  line L275 (14.3891, 6.1763) -> (14.1437, 5.9309)
  line L276 (14.1437, 4.2291) -> (14.3891, 3.9837)
  line L277 (14.1437, 5.9309) -> (13.7963, 5.9309)
  line L278 (72.6538, 12.1158) -> (72.3802, 12.1158)
  line L279 (4.8936, 6.7564) -> (5.241, 6.7564)
  line L280 (13.5509, 3.6363) -> (13.5509, 3.9837)
  line L281 (14.1437, 3.3909) -> (13.7963, 3.3909)
  line L282 (5.4864, 3.971) -> (5.4864, 3.6236)
  line L283 (13.7963, 3.3909) -> (13.5509, 3.6363)
  line L284 (13.5509, 3.6363) -> (13.5509, 3.9837)
  line L285 (4.6482, 6.511) -> (4.8936, 6.7564)
  line L286 (14.3891, 3.9837) -> (14.3891, 3.6363)
  line L287 (14.3891, 3.9837) -> (14.3891, 3.6363)
  line L288 (13.7963, 4.2291) -> (14.1437, 4.2291)
  line L289 (13.5509, 6.1763) -> (13.5509, 6.5237)
  line L290 (72.1868, 12.3092) -> (72.1868, 12.5828)
  line L291 (13.5509, 6.5237) -> (13.7963, 6.7691)
  line L292 (5.4864, 6.1636) -> (5.241, 5.9182)
  line L293 (13.7963, 3.3909) -> (13.5509, 3.6363)
  line L294 (14.3891, 3.6363) -> (14.1437, 3.3909)
  line L295 (14.1437, 6.7691) -> (14.3891, 6.5237)
  line L296 (13.7963, 6.7691) -> (14.1437, 6.7691)
  line L297 (5.241, 3.3782) -> (4.8936, 3.3782)
  line L298 (4.8936, 6.7564) -> (5.241, 6.7564)
  line L299 (13.7963, 5.9309) -> (13.5509, 6.1763)
  line L300 (13.7963, 6.7691) -> (14.1437, 6.7691)
  line L301 (14.3891, 6.5237) -> (14.3891, 6.1763)
  line L302 (13.7963, 4.2291) -> (14.1437, 4.2291)
  line L303 (13.7963, 5.9309) -> (13.5509, 6.1763)
  line L304 (5.241, 6.7564) -> (5.4864, 6.511)
  line L305 (13.7963, 6.7691) -> (14.1437, 6.7691)
  line L306 (4.8936, 4.2164) -> (5.241, 4.2164)
  line L307 (13.7963, 4.2291) -> (14.1437, 4.2291)
  line L308 (14.3891, 6.5237) -> (14.3891, 6.1763)
  line L309 (72.1868, 12.3092) -> (72.1868, 12.5828)
  line L310 (82.5402, 12.7762) -> (82.8138, 12.7762)
  line L311 (4.9686, 11.7475) -> (5.2422, 11.7475)
  line L312 (15.5956, 11.5541) -> (15.5956, 11.2805)
  line L313 (15.5956, 11.5541) -> (15.5956, 11.2805)
  line L314 (72.1868, 12.5828) -> (72.3802, 12.7762)
  line L315 (72.3802, 12.1158) -> (72.1868, 12.3092)
  line L316 (82.5402, 12.7762) -> (82.8138, 12.7762)
  line L317 (15.1286, 11.0871) -> (14.9352, 11.2805)
  line L318 (82.8138, 12.1158) -> (82.5402, 12.1158)
  line L319 (83.0072, 12.5828) -> (83.0072, 12.3092)
  line L320 (15.4022, 11.0871) -> (15.1286, 11.0871)
  line L321 (72.1868, 12.5828) -> (72.3802, 12.7762)
  line L322 (14.9352, 11.5541) -> (15.1286, 11.7475)
  line L323 (4.7752, 11.5541) -> (4.9686, 11.7475)
  line L324 (82.5402, 12.1158) -> (82.3468, 12.3092)
  line L325 (82.3468, 12.5828) -> (82.5402, 12.7762)
  line L326 (83.0072, 12.3092) -> (82.8138, 12.1158)
  line L327 (82.3468, 12.3092) -> (82.3468, 12.5828)
  line L328 (83.0072, 12.5828) -> (83.0072, 12.3092)
  line L329 (82.3468, 12.3092) -> (82.3468, 12.5828)
  line L330 (82.8138, 12.7762) -> (83.0072, 12.5828)
  line L331 (72.1868, 12.3092) -> (72.1868, 12.5828)
  line L332 (15.1286, 11.0871) -> (14.9352, 11.2805)
  line L333 (5.4356, 11.5541) -> (5.4356, 11.2805)
  line L334 (72.6538, 12.1158) -> (72.3802, 12.1158)
  line L335 (4.7752, 11.2805) -> (4.7752, 11.5541)
  line L336 (14.9352, 11.2805) -> (14.9352, 11.5541)
  line L337 (15.5956, 11.2805) -> (15.4022, 11.0871)
  line L338 (4.9686, 11.0871) -> (4.7752, 11.2805)
  line L339 (14.9352, 11.2805) -> (14.9352, 11.5541)
  line L340 (14.9352, 11.5541) -> (15.1286, 11.7475)
  line L341 (15.1286, 11.7475) -> (15.4022, 11.7475)
  line L342 (15.1286, 11.7475) -> (15.4022, 11.7475)
  line L343 (4.7752, 11.2805) -> (4.7752, 11.5541)
  line L344 (83.0072, 12.3092) -> (82.8138, 12.1158)
  line L345 (72.3802, 12.1158) -> (72.1868, 12.3092)
  line L346 (82.3468, 12.3092) -> (82.3468, 12.5828)
  line L347 (82.5402, 12.1158) -> (82.3468, 12.3092)
  line L348 (5.2422, 11.0871) -> (4.9686, 11.0871)
  line L349 (15.5956, 11.5541) -> (15.5956, 11.2805)
  line L350 (4.7752, 11.5541) -> (4.9686, 11.7475)
  line L351 (82.8138, 12.1158) -> (82.5402, 12.1158)
  line L352 (5.4356, 11.5541) -> (5.4356, 11.2805)
  line L353 (72.8472, 12.5828) -> (72.8472, 12.3092)
  line L354 (82.3468, 12.5828) -> (82.5402, 12.7762)
  line L355 (15.5956, 11.2805) -> (15.4022, 11.0871)
  line L356 (5.2422, 11.0871) -> (4.9686, 11.0871)
  line L357 (82.3468, 12.3092) -> (82.3468, 12.5828)
  line L358 (72.8472, 12.3092) -> (72.6538, 12.1158)
  line L359 (72.8472, 12.3092) -> (72.6538, 12.1158)
  line L360 (15.5956, 11.5541) -> (15.5956, 11.2805)
  line L361 (82.8138, 12.7762) -> (83.0072, 12.5828)
  line L362 (15.4022, 11.7475) -> (15.5956, 11.5541)
  line L363 (15.4022, 11.0871) -> (15.1286, 11.0871)
  line L364 (5.4356, 11.2805) -> (5.2422, 11.0871)
  line L365 (72.3802, 12.7762) -> (72.6538, 12.7762)
  line L366 (15.4022, 11.7475) -> (15.5956, 11.5541)
  line L367 (5.4356, 11.5541) -> (5.4356, 11.2805)
  line L368 (72.5268, 25.7302) -> (72.7202, 25.5368)
  line L369 (5.2422, 11.7475) -> (5.4356, 11.5541)
  line L370 (82.8802, 25.5368) -> (82.8802, 25.2632)
  line L371 (72.2532, 25.0698) -> (72.0598, 25.2632)
  line L372 (82.6868, 25.7302) -> (82.8802, 25.5368)
  line L373 (72.7202, 25.5368) -> (72.7202, 25.2632)
  line L374 (82.8802, 25.2632) -> (82.6868, 25.0698)
  line L375 (5.2422, 11.7475) -> (5.4356, 11.5541)
  line L376 (82.4132, 25.0698) -> (82.2198, 25.2632)
  line L377 (72.5268, 25.0698) -> (72.2532, 25.0698)
  line L378 (72.7202, 25.2632) -> (72.5268, 25.0698)
  line L379 (5.4356, 11.2805) -> (5.2422, 11.0871)
  line L380 (82.6868, 25.7302) -> (82.8802, 25.5368)
  line L381 (82.6868, 25.0698) -> (82.4132, 25.0698)
  line L382 (82.2198, 25.5368) -> (82.4132, 25.7302)
  line L383 (82.2198, 25.5368) -> (82.4132, 25.7302)
  line L384 (72.0598, 25.2632) -> (72.0598, 25.5368)
  line L385 (68.2498, 20.1832) -> (68.2498, 20.4568)
  line L386 (58.7502, 20.1832) -> (58.5568, 19.9898)
  line L387 (68.2498, 20.4568) -> (68.4432, 20.6502)
  line L388 (68.4432, 20.6502) -> (68.7168, 20.6502)
  line L389 (72.7202, 25.5368) -> (72.7202, 25.2632)
  line L390 (58.5568, 20.6502) -> (58.7502, 20.4568)
  line L391 (72.0598, 25.2632) -> (72.0598, 25.5368)
  line L392 (72.0598, 25.5368) -> (72.2532, 25.7302)
  line L393 (72.0598, 25.2632) -> (72.0598, 25.5368)
  line L394 (68.9102, 20.1832) -> (68.7168, 19.9898)
  line L395 (58.0898, 20.1832) -> (58.0898, 20.4568)
  line L396 (72.0598, 25.2632) -> (72.0598, 25.5368)
  line L397 (58.2832, 19.9898) -> (58.0898, 20.1832)
  line L398 (72.5268, 25.7302) -> (72.7202, 25.5368)
  line L399 (82.6868, 25.0698) -> (82.4132, 25.0698)
  line L400 (72.2532, 25.7302) -> (72.5268, 25.7302)
  line L401 (72.2532, 25.0698) -> (72.0598, 25.2632)
  line L402 (82.8802, 25.5368) -> (82.8802, 25.2632)
  line L403 (68.2498, 20.4568) -> (68.4432, 20.6502)
  line L404 (68.2498, 20.1832) -> (68.2498, 20.4568)
  line L405 (68.7168, 20.6502) -> (68.9102, 20.4568)
  line L406 (58.5568, 19.9898) -> (58.2832, 19.9898)
  line L407 (58.2832, 20.6502) -> (58.5568, 20.6502)
  line L408 (82.2198, 25.2632) -> (82.2198, 25.5368)
  line L409 (72.7202, 25.2632) -> (72.5268, 25.0698)
  line L410 (82.4132, 25.7302) -> (82.6868, 25.7302)
  line L411 (68.2498, 20.1832) -> (68.2498, 20.4568)
  line L412 (68.4432, 19.9898) -> (68.2498, 20.1832)
  line L413 (58.7502, 20.4568) -> (58.7502, 20.1832)
  line L414 (68.7168, 20.6502) -> (68.9102, 20.4568)
  line L415 (4.9686, 11.0871) -> (4.7752, 11.2805)
  line L416 (5.4356, 11.5541) -> (5.4356, 11.2805)
  line L417 (72.2532, 25.7302) -> (72.5268, 25.7302)
  line L418 (82.2198, 25.2632) -> (82.2198, 25.5368)
  line L419 (82.4132, 25.0698) -> (82.2198, 25.2632)
  line L420 (68.7168, 19.9898) -> (68.4432, 19.9898)
  line L421 (72.5268, 25.0698) -> (72.2532, 25.0698)
  line L422 (58.0898, 20.4568) -> (58.2832, 20.6502)
  line L423 (82.8802, 25.2632) -> (82.6868, 25.0698)
  line L424 (4.9686, 11.7475) -> (5.2422, 11.7475)
  line L425 (68.9102, 20.4568) -> (68.9102, 20.1832)
  line L426 (82.2198, 25.2632) -> (82.2198, 25.5368)
  line L427 (82.4132, 25.7302) -> (82.6868, 25.7302)
  line L428 (72.0598, 25.5368) -> (72.2532, 25.7302)
  line L429 (58.2832, 19.9898) -> (58.0898, 20.1832)
  line L430 (58.0898, 20.1832) -> (58.0898, 20.4568)
  line L431 (82.2198, 25.2632) -> (82.2198, 25.5368)
  line L432 (58.2832, 25.7302) -> (58.5568, 25.7302)
  line L433 (68.9102, 25.2632) -> (68.7168, 25.0698)
  line L434 (68.2498, 25.5368) -> (68.4432, 25.7302)
  line L435 (58.0898, 25.5368) -> (58.2832, 25.7302)
  line L436 (58.0898, 20.1832) -> (58.0898, 20.4568)
  line L437 (58.7502, 25.5368) -> (58.7502, 25.2632)
  line L438 (58.7502, 20.4568) -> (58.7502, 20.1832)
  line L439 (58.0898, 25.2632) -> (58.0898, 25.5368)
  line L440 (68.9102, 20.1832) -> (68.7168, 19.9898)
  line L441 (58.7502, 25.5368) -> (58.7502, 25.2632)
  line L442 (58.7502, 25.5368) -> (58.7502, 25.2632)
  line L443 (40.9702, 37.9632) -> (40.7768, 37.7698)
  line L444 (58.2832, 25.7302) -> (58.5568, 25.7302)
  line L445 (50.6632, 38.4302) -> (50.9368, 38.4302)
  line L446 (68.9102, 25.5368) -> (68.9102, 25.2632)
  line L447 (68.9102, 25.2632) -> (68.7168, 25.0698)
  line L448 (50.9368, 37.7698) -> (50.6632, 37.7698)
  line L449 (40.7768, 38.4302) -> (40.9702, 38.2368)
  line L450 (51.1302, 38.2368) -> (51.1302, 37.9632)
  line L451 (50.4698, 37.9632) -> (50.4698, 38.2368)
  line L452 (40.9702, 38.2368) -> (40.9702, 37.9632)
  line L453 (40.7768, 37.7698) -> (40.5032, 37.7698)
  line L454 (68.9102, 25.5368) -> (68.9102, 25.2632)
  line L455 (68.2498, 25.5368) -> (68.4432, 25.7302)
  line L456 (58.5568, 25.7302) -> (58.7502, 25.5368)
  line L457 (58.0898, 20.4568) -> (58.2832, 20.6502)
  line L458 (50.9368, 38.4302) -> (51.1302, 38.2368)
  line L459 (58.5568, 19.9898) -> (58.2832, 19.9898)
  line L460 (40.7768, 37.7698) -> (40.5032, 37.7698)
  line L461 (58.5568, 25.0698) -> (58.2832, 25.0698)
  line L462 (68.7168, 19.9898) -> (68.4432, 19.9898)
  line L463 (40.5032, 37.7698) -> (40.3098, 37.9632)
  line L464 (40.5032, 38.4302) -> (40.7768, 38.4302)
  line L465 (40.3098, 37.9632) -> (40.3098, 38.2368)
  line L466 (58.2832, 25.0698) -> (58.0898, 25.2632)
  line L467 (68.2498, 25.2632) -> (68.2498, 25.5368)
  line L468 (50.6632, 38.4302) -> (50.9368, 38.4302)
  line L469 (68.9102, 25.5368) -> (68.9102, 25.2632)
  line L470 (68.7168, 25.0698) -> (68.4432, 25.0698)
  line L471 (68.7168, 25.0698) -> (68.4432, 25.0698)
  line L472 (68.7168, 25.7302) -> (68.9102, 25.5368)
  line L473 (58.7502, 20.1832) -> (58.5568, 19.9898)
  line L474 (58.2832, 20.6502) -> (58.5568, 20.6502)
  line L475 (58.0898, 25.5368) -> (58.2832, 25.7302)
  line L476 (68.4432, 25.7302) -> (68.7168, 25.7302)
  line L477 (58.7502, 25.5368) -> (58.7502, 25.2632)
  line L478 (68.9102, 20.4568) -> (68.9102, 20.1832)
  line L479 (68.4432, 20.6502) -> (68.7168, 20.6502)
  line L480 (58.0898, 25.2632) -> (58.0898, 25.5368)
  line L481 (68.2498, 25.2632) -> (68.2498, 25.5368)
  line L482 (68.4432, 25.7302) -> (68.7168, 25.7302)
  line L483 (58.5568, 25.7302) -> (58.7502, 25.5368)
  line L484 (68.4432, 25.0698) -> (68.2498, 25.2632)
  line L485 (58.2832, 25.0698) -> (58.0898, 25.2632)
  line L486 (58.7502, 25.2632) -> (58.5568, 25.0698)
  line L487 (58.5568, 25.0698) -> (58.2832, 25.0698)
  line L488 (68.9102, 25.5368) -> (68.9102, 25.2632)
  line L489 (58.7502, 25.2632) -> (58.5568, 25.0698)
  line L490 (68.4432, 19.9898) -> (68.2498, 20.1832)
  line L491 (68.2498, 20.1832) -> (68.2498, 20.4568)
  line L492 (58.0898, 20.1832) -> (58.0898, 20.4568)
  line L493 (58.5568, 20.6502) -> (58.7502, 20.4568)
  line L494 (68.4432, 25.0698) -> (68.2498, 25.2632)
  line L495 (68.7168, 25.7302) -> (68.9102, 25.5368)
  line L496 (51.1302, 42.0468) -> (51.1302, 41.7732)
  line L497 (50.9368, 42.2402) -> (51.1302, 42.0468)
  line L498 (40.7768, 42.2402) -> (40.9702, 42.0468)
  line L499 (50.6632, 37.7698) -> (50.4698, 37.9632)
  line L500 (40.3098, 41.7732) -> (40.3098, 42.0468)
  line L501 (51.1302, 41.7732) -> (50.9368, 41.5798)
  line L502 (51.1302, 41.7732) -> (50.9368, 41.5798)
  line L503 (40.9702, 37.9632) -> (40.7768, 37.7698)
  line L504 (40.9702, 38.2368) -> (40.9702, 37.9632)
  line L505 (50.9368, 38.4302) -> (51.1302, 38.2368)
  line L506 (50.9368, 42.2402) -> (51.1302, 42.0468)
  line L507 (40.7768, 41.5798) -> (40.5032, 41.5798)
  line L508 (50.9368, 41.5798) -> (50.6632, 41.5798)
  line L509 (40.9702, 41.7732) -> (40.7768, 41.5798)
  line L510 (50.6632, 37.7698) -> (50.4698, 37.9632)
  line L511 (50.4698, 38.2368) -> (50.6632, 38.4302)
  line L512 (40.3098, 38.2368) -> (40.5032, 38.4302)
  line L513 (51.1302, 37.9632) -> (50.9368, 37.7698)
  line L514 (40.5032, 42.2402) -> (40.7768, 42.2402)
  line L515 (40.9702, 42.0468) -> (40.9702, 41.7732)
  line L516 (36.4998, 41.7732) -> (36.4998, 42.0468)
  line L517 (50.4698, 37.9632) -> (50.4698, 38.2368)
  line L518 (36.4998, 41.7732) -> (36.4998, 42.0468)
  line L519 (40.9702, 42.0468) -> (40.9702, 41.7732)
  line L520 (40.9702, 38.2368) -> (40.9702, 37.9632)